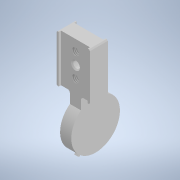
# Autodesk Inventor part: 1310162 DHRS-25-A---(Griff)
Saved by Autodesk Inventor 2021 (Build 250183000, 183)
## iProperties
Created: 2025-06-13
Part Number: 1310162 DHRS-25-A---(Griff)
Material: Generic
Catalog Web Link: www.cadenas.de
Description: DHRS---(Griff)-Handle
Vendor: FESTO
Document SubType Name: Modeling
Designer: psAdmin
Manufacturer: FESTO
Mass: 3.83337 g
Surface Area: 24.7736 cm^2
Volume: 3.83337 cm^3
Density: 1 g/cm^3
Appearance: PSOLRGB-175-175-175
Category: PARTsolutions
Company: FESTO
Title: 1310162 DHRS-25-A---(Griff)
Author: Cadenas PARTsolutions
Comments: Handle
PSOL_IDENT_0: {$CADENAS_DATA/23d-libs/festo/parts/d/dhrs/parts/dhrs_griff.prj},202 {VTYP=3D},{NB=1310162 DHRS-25-A
PSOL_IDENT_1: ---(Griff)},{LINA=1310162 DHRS-25-A---(Griff)},{NN=DHRS---(Griff)},{DATE=04.06.2025 19:34:44},{GEOMD
PSOL_IDENT_2: ATE=22.08.2023 11:13:58},{VERSION=},{LINEID=40},{WBVAR=},{WBNUMERIC=}  {NB=1310162 DHRS-25-A---(Grif
PSOL_IDENT_3: f)},{LINA=1310162 DHRS-25-A---(Griff)},{KT=DUMMY},{TNR=1310162},{TYP=DHRS-25-A},{GR=25}
NB: 1310162 DHRS-25-A---(Griff)
NN: DHRS---(Griff)
NT: Handle
NBSYN: $TNR. $TYP.---(Griff)
LINA: 1310162 DHRS-25-A---(Griff)
CATALOG: Festo
TNR: 1310162
TYP: DHRS-25-A
GR: 25
SUPPLIER: FESTO
ARTICLENO: 1310162 DHRS-25-A---(Griff)
BOMINFO: 1310162 DHRS-25-A---(Griff)
CREATOR: CADENAS GmbH
Autodesk Inventor part; units mm, degrees
sketch "Sketch_1" plane through (0, 0, 0) normal (1, 0, 0) x (0, 1, 0)
  arc A0 (8.7499, 6.5) -> (10.8427, -1.1157) centre (0, 0) ccw
  arc A1 (12.6333, 0.5) -> (10.8427, -1.1157) centre (12.6333, -1.3) ccw
  line L0 (12.6333, 0.5) -> (35.2, 0.5)
  line L1 (35.2, 0.5) -> (35.2, 6.5)
  line L2 (35.2, 6.5) -> (8.7499, 6.5)
  constraints: 6 end point, 4 point on circle, 2 centre point
extrude "Extrusion1" add sketch "Sketch_1" along normal mid plane 13
sketch "Sketch_2" plane through (0, 0, 0) normal (0, 0, 1) x (1, 0, 0)
  line L0 (-6.5, -21.8) -> (6.5, -21.8)
  line L1 (6.5, -21.8) -> (6.5, 14)
  line L2 (6.5, 14) -> (3.5, 14)
  arc A0 (3.5, 14) -> (2.5, 13) centre (3.5, 13) ccw
  line L3 (2.5, 13) -> (2.5, -18.8)
  line L4 (2.5, -18.8) -> (-2.5, -18.8)
  line L5 (-2.5, -18.8) -> (-2.5, 13)
  arc A1 (-2.5, 13) -> (-3.5, 14) centre (-3.5, 13) ccw
  line L6 (-3.5, 14) -> (-6.5, 14)
  line L7 (-6.5, 14) -> (-6.5, -21.8)
  constraints: 16 end point, 4 point on circle, 2 centre point
extrude "Extrusion2" cut sketch "Sketch_2" along normal mid plane 30
sketch "Sketch_3" plane through (0, 0, 7.5) normal (0, 0, 1) x (1, 0, 0)
  line L0 (6.5, 14) -> (7, 14)
  line L1 (7, 14) -> (7.5, 14.5)
  line L2 (7.5, 14.5) -> (7.5, 34.7)
  line L3 (7.5, 34.7) -> (7, 35.2)
  line L4 (7, 35.2) -> (6.5, 35.2)
  line L5 (6.5, 35.2) -> (6.5, 14)
  constraints: 12 end point
extrude "Extrusion3" add sketch "Sketch_3" against normal blind 8
sketch "Sketch_4" plane through (0, 0, 7.5) normal (0, 0, 1) x (1, 0, 0)
  line L0 (-7.5, 14.5) -> (-7, 14)
  line L1 (-7, 14) -> (-6.5, 14)
  line L2 (-6.5, 14) -> (-6.5, 35.2)
  line L3 (-6.5, 35.2) -> (-7, 35.2)
  line L4 (-7, 35.2) -> (-7.5, 34.7)
  line L5 (-7.5, 34.7) -> (-7.5, 14.5)
  constraints: 12 end point
extrude "Extrusion4" add sketch "Sketch_4" against normal blind 8
sketch "Sketch_5" plane through (0, 0, 0) normal (1, 0, 0) x (0, 1, 0)
  line L0 (24.95, 0.5) -> (24.95, 6.5)
  line L1 (24.95, 6.5) -> (26.95, 6.5)
  line L2 (26.95, 6.5) -> (26.45, 6)
  line L3 (26.45, 6) -> (26.45, 1)
  line L4 (26.45, 1) -> (26.95, 0.5)
  line L5 (26.95, 0.5) -> (24.95, 0.5)
  line L6 (24.95, 0.5) -> (24.95, 6.5)
  constraints: 14 end point
revolve "Revolution1" cut sketch "Sketch_5" angle 360 about axis through (0, 24.95, 0.5) along (0, 0, -1)
sketch "Sketch6" plane through (-2.5, 8.7499, 6.5) normal (0, 0, 1) x (1, 0, 0)
  point P0 (2.5, 10.9501)
hole "Hole1" at (0, 19.7, 6.5) direction (0, 0, -1) diameter 3.242 depth 6 thread size "M4x0.7" class "6H" standard "ISO Metric profile"
sketch "Sketch7" plane through (-2.5, 8.7499, 6.5) normal (0, 0, 1) x (1, 0, 0)
  point P0 (2.5, 21.4501)
hole "Hole2" at (0, 30.2, 6.5) direction (0, 0, -1) diameter 3.242 depth 6 thread size "M4x0.7" class "6H" standard "ISO Metric profile"
sketch "Sketch_9" plane through (0, 0, 0) normal (1, 0, 0) x (0, 1, 0)
  arc A0 (-10.0918, 6.306) -> (-10.603, 5.4025) centre (0, 0) ccw
  line L0 (-10.603, 5.4025) -> (0, 0)
  line L1 (0, 0) -> (-10.0918, 6.306)
  constraints: 4 end point, 2 point on circle, 1 centre point
extrude "Extrusion5" add sketch "Sketch_9" along normal mid plane 1.5
ref_plane "GRIFF_XY" through (0, 0, 0) normal (1, 0, 0) x (0, 0, -1)
ref_plane "GRIFF_YZ" through (0, 0, 0) normal (0, 0, -1) x (0, 1, 0)
ref_plane "GRIFF_ZX" through (0, 0, 0) normal (0, 1, 0) x (1, 0, 0)
body "Solid1"
